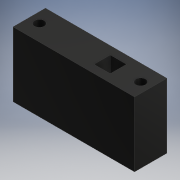
# Autodesk Inventor part: SupportPlateau
Saved by Autodesk Inventor 2017 (Build 210142000, 142)
## iProperties
Created: 2017-10-26
Part Number: SupportPlateau
Material: PC/ABS Plastic
Document SubType Name: Modeling
Designer: Biscuit
Density: 0.357273 g/cm^3
Appearance: Glossy - Black
Author: Biscuit
Autodesk Inventor part; units mm, degrees
ref_plane "YZ Plane" through (0, 0, 0) normal (1, 0, 0) x (0, 1, 0)
ref_plane "XZ Plane" through (0, 0, 0) normal (0, 1, 0) x (-1, 0, 0)
ref_plane "XY Plane" through (0, 0, 0) normal (0, 0, 1) x (1, 0, 0)
sketch "Sketch3" plane through (0, 0, 0) normal (0, 0, 1) x (1, 0, 0)
  line L0 (0, 0) -> (75, 0)
  line L1 (75, 0) -> (75, 20)
  line L2 (75, 20) -> (0, 20)
  line L3 (0, 20) -> (0, 0)
  circle A0 centre (6.25, 10) radius 3
  circle A1 centre (68.75, 10) radius 3
  line L4 (45, 15) -> (55, 15)
  line L5 (55, 15) -> (55, 5)
  line L6 (55, 5) -> (45, 5)
  line L7 (45, 5) -> (45, 15)
  dimension "d19" = 20
  dimension "d20" = 75
  dimension "d21" = 6
  dimension "d22" = 6
  dimension "d23" = 10
  dimension "d24" = 10
  dimension "d25" = 62.5
  dimension "d26" = 6.25
  dimension "d30" = 10
  dimension "d31" = 10
  dimension "d32" = 5
  dimension "d33" = 20
  constraints: 16 end point, 4 parallel, 2 centre point, 2 horizontal, 2 perpendicular
  measures "d19" distance of L2.end L0.start
  measures "d20" distance of L1.end L2.end
  measures "d21" diameter of A0
  measures "d22" diameter of A1
  measures "d23" distance from line of L0 A0.centre
  measures "d24" distance from line of L0 A1.centre
  measures "d25" distance of A1.centre A0.centre
  measures "d26" distance from line of L3 A0.centre
  measures "d30" distance of L6.end L4.start
  measures "d31" distance of L4.start L4.end
  measures "d32" distance between parallel lines of L2 L4
  measures "d33" distance between parallel lines of L1 L5
extrude "Extrusion3" add sketch "Sketch3" along normal blind 40
equation "\"d22\" = d21"
equation "\"d23\" = 0.5 * d19"
equation "\"d24\" = 0.5 * d19"
equation "\"d26\" = 0.5 * d20 - 0.5 * d25"
body "Solid2"
